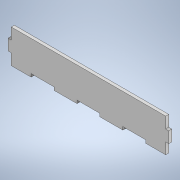
# Autodesk Inventor part: back
Saved by Autodesk Inventor 2020 (Build 240168000, 168)
## iProperties
Created: 2020-02-22
Part Number: back
Material: Generic
Document SubType Name: Modeling
Designer: udvarhelyi
Density: 1 g/cm^3
Appearance: Default
Author: udvarhelyi
Autodesk Inventor part; units mm, degrees
ref_plane "YZ Plane" through (0, 0, 0) normal (1, 0, 0) x (0, 1, 0)
ref_plane "XZ Plane" through (0, 0, 0) normal (0, 1, 0) x (-1, 0, 0)
ref_plane "XY Plane" through (0, 0, 0) normal (0, 0, 1) x (1, 0, 0)
sketch "Sketch1" plane through (0, 0, 0) normal (0, 0, 1) x (1, 0, 0)
  line L0 (-33.8571, 0) -> (-33.8571, 3)
  line L1 (-33.8571, 3) -> (-56.4286, 3)
  line L2 (-56.4286, 3) -> (-56.4286, 0)
  line L3 (11.2857, 0) -> (11.2857, 3)
  line L4 (11.2857, 3) -> (-11.2857, 3)
  line L5 (-11.2857, 3) -> (-11.2857, 0)
  line L6 (56.4286, 0) -> (56.4286, 3)
  line L7 (56.4286, 3) -> (33.8571, 3)
  line L8 (33.8571, 3) -> (33.8571, 0)
  line L9 (-79, 22) -> (-79, 22)
  line L10 (-79, 22) -> (-79, 11)
  line L11 (-79, 11) -> (-79, 11)
  line L12 (79, 11) -> (79, 11)
  line L13 (79, 11) -> (79, 22)
  line L14 (79, 22) -> (79, 22)
  line L15 (-56.4286, 33) -> (-79, 33)
  line L16 (79, 33) -> (56.4286, 33)
  line L17 (33.8571, 33) -> (11.2857, 33)
  line L18 (-11.2857, 33) -> (-33.8571, 33)
  line L19 (79, 0) -> (79, 11)
  line L20 (79, 22) -> (79, 33)
  line L21 (56.4286, 0) -> (79, 0)
  line L22 (11.2857, 0) -> (33.8571, 0)
  line L23 (-79, 0) -> (-56.4286, 0)
  line L24 (-33.8571, 0) -> (-11.2857, 0)
  line L25 (-79, 33) -> (-79, 22)
  line L26 (-79, 11) -> (-79, 0)
  line L27 (-56.4286, 33) -> (57.8569, 33)
  point P0 (0, 0)
  point P1 (0, 30)
  point P2 (52.5, 33)
  dimension "d46" = 158
  dimension "d48" = 33
  dimension "d49" = 79
  dimension "d50" = 0
  dimension "d53" = 0
  dimension "d58" = 11
  dimension "d59" = 11
  dimension "d61" = 22.5714
  dimension "d62" = 11.2857
  dimension "d63" = 0
  dimension "d64" = 0
  dimension "d65" = 3
  constraints: 56 end point, 25 parallel, 11 perpendicular, 10 collinear, 8 equal length, 8 point on line, 6 horizontal, 1 other
  measures "d46" distance of L16.start L15.end
  measures "d48" distance between parallel lines of L21 L16
  measures "d49" distance from line of L20 point (0, 0)
  measures "d50" distance from line of L21 point (0, 0)
  measures "d53" horizontal distance of point (0, 0) point (0, 30)
  measures "d58" distance of L15.end L9.start
  measures "d59" distance of L9.end L10.end
  measures "d61" distance of L0.start L5.end
  measures "d62" distance from line of L5 point (0, 0)
  measures "d63" distance of L9.start L9.end
  measures "d64" distance of L13.end L14.end
  measures "d65" distance of L1.end L2.end
extrude "Extrusion1" add sketch "Sketch1" along normal blind 3
sketch "Sketch3" plane through (0, 0, 3) normal (0, 0, 1) x (1, 0, 0)
  line L0 (-79, 33) -> (-79, 0) projected
  line L1 (-79, 33) -> (-76, 33)
  line L2 (-76, 33) -> (-76, 22)
  line L3 (-76, 22) -> (-79, 22)
  line L4 (-79, 22) -> (-79, 33)
  line L5 (-79, 0) -> (-56.4286, 0) projected
  line L6 (-79, 0) -> (-76, 0)
  line L7 (-76, 0) -> (-76, 11)
  line L8 (-76, 11) -> (-79, 11)
  line L9 (-79, 11) -> (-79, 0)
  line L10 (79, 33) -> (-79, 33) projected
  line L11 (79, 33) -> (76, 33)
  line L12 (76, 33) -> (76, 22)
  line L13 (76, 22) -> (79, 22)
  line L14 (79, 22) -> (79, 33)
  line L15 (79, 0) -> (79, 33) projected
  line L16 (79, 0) -> (76, 0)
  line L17 (76, 0) -> (76, 11)
  line L18 (76, 11) -> (79, 11)
  line L19 (79, 11) -> (79, 0)
  point P0 (0, 0)
  dimension "d66" = 11
  dimension "d67" = 3
  constraints: 32 end point, 8 parallel, 4 horizontal, 4 perpendicular, 4 point on line, 2 collinear
  measures "d66" distance of L1.end L2.end
  measures "d67" distance of L2.end L3.end
extrude "Extrusion3" cut sketch "Sketch3" against normal through all
equation "\"d46\" = shelfWs"
equation "\"d48\" = shelfD"
equation "\"d49\" = 0.5 * shelfWs"
equation "\"d58\" = 0.333333 * shelfD - tol"
equation "\"d59\" = 0.333333 * shelfD + 2 * tol"
equation "\"d24\" = tt"
equation "\"d0\" = 0.5 * shelfWs"
equation "\"tt\" = 3"
equation "\"tol\" = 0"
equation "\"d2\" = shelfD"
equation "\"d4\" = tt"
equation "\"tiroir\" = 1"
equation "\"nHoles\" = 4"
equation "\"shelfH\" = 35"
equation "\"shelfWs\" = 158"
equation "\"d47\" = 0.5 * shelfWs"
equation "\"shelfD\" = 33"
body "Solid1"
